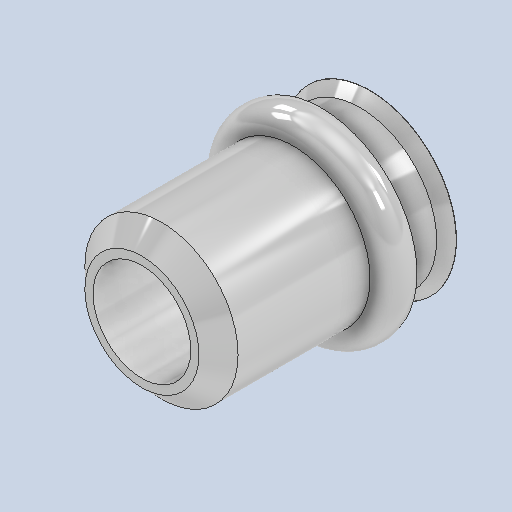
# Autodesk Inventor part: pop_PSZROX-0315
Saved by Autodesk Inventor 2022 (Build 260153000, 153)
## iProperties
Created: 2020-06-16
Part Number: pop_PSZROX-0315
Material: Generic
Document SubType Name: Modeling
Designer: Viktor Lindström
Density: 1 g/cm^3
Appearance: Default
Author: Viktor Lindström
Autodesk Inventor part; units mm, degrees
ref_plane "YZ Plane" through (0, 0, 0) normal (1, 0, 0) x (0, 1, 0)
ref_plane "XZ Plane" through (0, 0, 0) normal (0, 1, 0) x (-1, 0, 0)
sketch "Sketch1" plane through (0, 0, 0) normal (0, 0, 1) x (1, 0, 0)
  circle A0 centre (0, 0) radius 2.35
  dimension "d0" = 4.7
  constraints: 1 centre point, 1 coincident
  measures "d0" diameter of A0
extrude "Extrusion1" add sketch "Sketch1" along normal blind 7
chamfer "Chamfer1" distance 0.6 angle 45 1 edges at (-2.35, 0, 7)
sketch "Sketch2" plane through (0, 0, 0) normal (0, 0, -1) x (-1, 0, 0)
  circle A0 centre (0, 0) radius 1.5
  dimension "d6" = 3
  constraints: 1 centre point, 1 coincident
  measures "d6" diameter of A0
extrude "Extrusion2" cut sketch "Sketch2" against normal through all
sketch "Sketch3" plane through (0, 0, 0) normal (0, 0, -1) x (-1, 0, 0)
  circle A0 centre (0, 0) radius 2.65
  dimension "d11" = 5.3
  constraints: 1 centre point, 1 coincident
  measures "d11" diameter of A0
extrude "Extrusion3" add sketch "Sketch3" against normal blind 0.01
chamfer "Chamfer2" distance 0.3 angle 45 1 edges at (-2.35, 0, 0.01)
sketch "Sketch4" plane through (0, 0, 0.01) normal (0, 0, 1) x (1, 0, 0)
  circle A0 centre (0, 0) radius 1.5 projected
extrude "Extrusion4" cut sketch "Sketch4" against normal through all
ref_plane "Work Plane1" through (0, 0, 1.5) normal (0, 0, -1) x (-1, 0, 0)
sketch "Sketch5" plane through (0, 0, 1.5) normal (0, 0, -1) x (-1, 0, 0)
  circle A0 centre (0, 0) radius 2.35 projected
  circle A1 centre (0, 0) radius 2.35 projected
sketch "Sketch6" plane through (0, 0, 0) normal (1, 0, 0) x (0, 1, 0)
  line L0 (2.35, 0.31) -> (2.35, 6.4) projected
  line L1 (3.71, 1.5) -> (-3.71, 1.5) projected
  circle A0 centre (2.4109, 1.7672) radius 0.5891
  line L2 (2.9359, 1.5) -> (2.35, 1.5)
  line L3 (2.35, 1.5) -> (2.35, 2.3531)
  line L4 (0, -1.4) -> (0, 8.4) projected
  point P0 (0, 0)
  dimension "d18" = 3
  constraints: 4 end point, 4 point on line, 2 point on circle, 1 centre point
sweep "Sweep1" add profiles "Sketch6" path "Sketch5" picked at (2.489, 2.0554) path curves A0 contours L0 A0 L1
body "Solid1"
